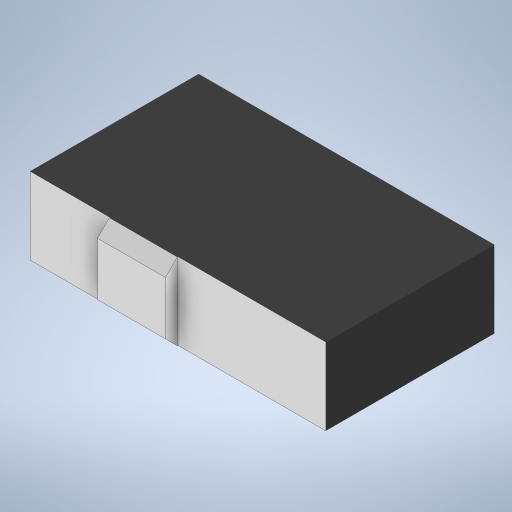
# Autodesk Inventor part: wlacznik
Saved by Autodesk Inventor 2023 (Build 270158000, 158)
## iProperties
Created: 2023-08-22
Part Number: wlacznik
Material: Ogólny
Document SubType Name: Modeling
Designer: Kamil
Density: 1 g/cm^3
Appearance: Domyślna
Author: Kamil
Autodesk Inventor part; units mm, degrees
ref_plane "YZ Plane" through (0, 0, 0) normal (1, 0, 0) x (0, 1, 0)
ref_plane "XZ Plane" through (0, 0, 0) normal (0, 1, 0) x (-1, 0, 0)
ref_plane "XY Plane" through (0, 0, 0) normal (0, 0, 1) x (1, 0, 0)
sketch "Szkic1" plane through (0, 0, 0) normal (0, 1, 0) x (-1, 0, 0)
  line L0 (0, 0) -> (10, 0)
  line L1 (10, 0) -> (10, -5.7)
  line L2 (10, -5.7) -> (0, -5.7)
  line L3 (0, -5.7) -> (0, 0)
  dimension "d0" = 10
  dimension "d1" = 5.7
  constraints: 8 end point, 2 parallel, 1 horizontal, 1 perpendicular
  measures "d0" distance of L1.end L2.end
  measures "d1" distance of L0.end L1.end
extrude "Wyciągnięcie proste1" add sketch "Szkic1" along normal blind 2.6
sketch "Szkic2" plane through (-10, 0, 0) normal (0, 0, 1) x (1, 0, 0)
  line L0 (0, 0) -> (10, 0) projected
  line L1 (10, 0) -> (10, 2.6) projected
  line L2 (0, 2.6) -> (10, 2.6) projected
  line L3 (0, 0) -> (0, 2.6) projected
  line L4 (0, 0) -> (0, 2.6) projected
  line L5 (10, 0) -> (0, 0) projected
  line L6 (0, 2.6) -> (2.7, 2.6)
  line L7 (2.7, 2.6) -> (2.7, 0)
  line L8 (2.7, 0) -> (0, 0)
  line L9 (0, 0) -> (0, 2.6)
  line L10 (10, 2.6) -> (0, 2.6) projected
  line L11 (2.7, 0) -> (5, 0)
  line L12 (5, 0) -> (5, 2.6)
  line L13 (5, 2.6) -> (2.7, 2.6)
  line L14 (2.7, 2.6) -> (2.7, 0)
  dimension "d4" = 2.7
  constraints: 16 end point, 4 parallel, 2 horizontal, 2 perpendicular, 1 midpoint, 1 point on line
  measures "d4" distance of L7.end L8.end
extrude "Wyciągnięcie proste2" add sketch "Szkic2" along normal blind 0.42 contours L7 L2 L12 L0
chamfer "Faza1" distance 0.4 angle 45 2 edges at (-6.15, 2.6, 0.42) (-6.15, 0, 0.42)
